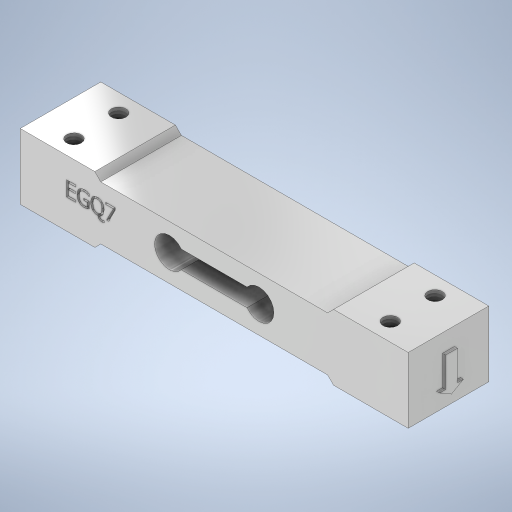
# Autodesk Inventor part: HCMUTE-CDT23-LOADCELL
Saved by Autodesk Inventor 2023 (Build 270158000, 158)
## iProperties
Created: 2023-10-10
Part Number: HCMUTE-CDT23-LOADCELL
Material: Aluminum 6061
Document SubType Name: Modeling
Designer: havie
Density: 2.7 g/cm^3
Appearance: Aluminum - Polished
Author: havie
Autodesk Inventor part; units mm, degrees
note: some values were not read from the file. Chosen so that the rebuilt part matches the saved one: direction of "Emboss1".
ref_plane "YZ Plane" through (0, 0, 0) normal (1, 0, 0) x (0, 1, 0)
ref_plane "XZ Plane" through (0, 0, 0) normal (0, 1, 0) x (-1, 0, 0)
ref_plane "XY Plane" through (0, 0, 0) normal (0, 0, 1) x (1, 0, 0)
sketch "Sketch1" plane through (0, 0, 0) normal (0, 0, 1) x (1, 0, 0)
  line L0 (-65, -13.5) -> (65, -13.5)
  line L1 (65, -13.5) -> (65, 13.5)
  line L2 (65, 13.5) -> (-65, 13.5)
  line L3 (-65, 13.5) -> (-65, -13.5)
  line L4 (-65, -13.5) -> (65, 13.5) construction
  line L5 (65, -13.5) -> (-65, 13.5) construction
  point P0 (0, 0)
  dimension "d0" = 27
  dimension "d1" = 130
  constraints: 12 end point, 2 midpoint, 2 parallel, 1 horizontal, 1 perpendicular
  measures "d0" distance between parallel lines of L2 L0
  measures "d1" distance of L1.end L2.end
extrude "Extrusion1" add sketch "Sketch1" along normal mid plane 22
sketch "Sketch2" plane through (0, 0, 11) normal (0, 0, 1) x (1, 0, 0)
  line L0 (-65, -13.5) -> (65, -13.5) projected
  line L1 (65, -13.5) -> (65, 13.5) projected
  line L2 (-65, 13.5) -> (-65, -13.5) projected
  point P0 (0, 0)
  point P1 (-53, -7.5)
  point P2 (-53, 7.5)
  point P3 (53, 7.5)
  point P4 (53, -7.5)
  dimension "d4" = 6
  dimension "d5" = 15
  dimension "d6" = 12
  dimension "d7" = 12
  constraints: 2 horizontal alignment, 2 vertical alignment
  measures "d4" distance from line of point (53, -7.5) L0
  measures "d5" distance of point (53, 7.5) point (53, -7.5)
  measures "d6" distance from line of L1 point (53, -7.5)
  measures "d7" distance from line of point (-53, -7.5) L2
hole "Hole1" at (-53, -7.5, 11) at (-53, 7.5, 11) at (53, 7.5, 11) at (53, -7.5, 11) direction (0, 0, -1) diameter 4.917 end through all thread size "M6x1" class "6H" standard "ISO Metric profile"
sketch "Sketch3" plane through (-65, -13.5, 11) normal (0, -1, 0) x (1, 0, 0)
  line L0 (0, 0) -> (130, 0) projected
  line L1 (25, 0) -> (27, -2)
  line L2 (27, -2) -> (103, -2)
  line L3 (103, -2) -> (105, 0)
  point P0 (65, -11)
  dimension "d15" = 25
  dimension "d16" = 25
  dimension "d17" = 2
  dimension "d18" = 135
  constraints: 6 end point, 2 point on line, 1 parallel, 1 perpendicular
  measures "d15" distance of L0.start L1.start
  measures "d16" distance of L3.end L0.end
  measures "d17" distance between parallel lines of L0 L2
  measures "d18" angle of L2 L1
extrude "Extrusion2" cut sketch "Sketch3" against normal through all
mirror "Mirror1" about plane through (0, 0, 0) normal (0, 0, 1) of "Extrusion2"
sketch "Sketch4" plane through (65, -13.5, -11) normal (0, -1, 0) x (1, 0, 0)
  circle A0 centre (-80, 11) radius 5
  circle A1 centre (-50, 11) radius 5
  line L0 (-25, 22) -> (0, 22) projected
  line L1 (-76, 14) -> (-54, 14)
  line L2 (-76, 8) -> (-54, 8)
  point P0 (-65, 11)
  dimension "d21" = 10
  dimension "d22" = 10
  dimension "d23" = 30
  dimension "d24" = 15
  dimension "d25" = 11
  dimension "d26" = 6
  dimension "d27" = 3
  constraints: 4 end point, 4 point on circle, 2 centre point, 2 horizontal, 1 horizontal alignment
  measures "d21" diameter of A0
  measures "d22" diameter of A1
  measures "d23" distance of A1.centre A0.centre
  measures "d24" distance of point (-65, 11) A0.centre
  measures "d25" distance from line of L0 A1.centre
  measures "d26" distance between parallel lines of L2 L1
  measures "d27" distance from line of L1 point (-65, 11)
extrude "Extrusion3" cut sketch "Sketch4" against normal through all
sketch "Sketch5" plane through (65, -13.5, 11) normal (1, 0, 0) x (0, 0, -1)
  line L0 (6, 11.5) -> (16, 11.5)
  line L1 (16, 11.5) -> (16, 15.5)
  line L2 (16, 15.5) -> (6, 15.5)
  line L3 (6, 15.5) -> (6, 11.5)
  line L4 (16, 0) -> (16, 27) projected
  line L5 (16, 9.5) -> (18.3094, 13.5)
  line L6 (18.3094, 13.5) -> (16, 17.5)
  line L7 (16, 9.5) -> (16, 17.5)
  point P0 (11, 13.5)
  point P1 (11, 15.5)
  point P2 (16, 11.5)
  dimension "d30" = 4
  dimension "d31" = 2
  dimension "d32" = 10
  dimension "d33" = 5
  dimension "d34" = 8
  dimension "d35" = 2
  dimension "d36" = 30
  constraints: 14 end point, 2 parallel, 2 point on line, 1 collinear, 1 horizontal, 1 horizontal alignment, 1 midpoint, 1 perpendicular
  measures "d30" distance from line of point (11, 15.5) L0
  measures "d31" distance from line of L0 point (11, 13.5)
  measures "d32" distance of L1.end L2.end
  measures "d33" distance from line of point (11, 13.5) L3
  measures "d34" distance of L5.start L6.end
  measures "d35" distance from line of L6.end L2
  measures "d36" angle of L1 L5
extrude "Extrusion4" add sketch "Sketch5" along normal blind 1
sketch "Sketch6" plane through (65, -13.5, -11) normal (0, -1, 0) x (1, 0, 0)
  line L0 (-115, 15) -> (-100, 15) construction
  line L1 (-100, 15) -> (-100, 5) construction
  line L2 (-100, 5) -> (-115, 5) construction
  line L3 (-115, 5) -> (-115, 15) construction
  line L4 (-130, 0) -> (-130, 22) projected
  line L5 (-105, 0) -> (-130, 0) projected
  line L6 (-114.4935, 9.8947) -> (-114.4935, 14.8947)
  line L7 (-114.4935, 14.8947) -> (-111.3655, 14.8947)
  line L8 (-111.3655, 14.8947) -> (-111.3655, 14.3031)
  line L9 (-111.3655, 14.3031) -> (-113.829, 14.3031)
  line L10 (-113.829, 14.3031) -> (-113.829, 12.9335)
  line L11 (-113.829, 12.9335) -> (-111.5316, 12.9335)
  line L12 (-111.5316, 12.9335) -> (-111.5316, 12.342)
  line L13 (-111.5316, 12.342) -> (-113.829, 12.342)
  line L14 (-113.829, 12.342) -> (-113.829, 10.4862)
  line L15 (-113.829, 10.4862) -> (-111.3655, 10.4862)
  line L16 (-111.3655, 10.4862) -> (-111.3655, 9.8947)
  line L17 (-111.3655, 9.8947) -> (-114.4935, 9.8947)
  spline S0 degree 2 poles (-108.5413, 9.7974) (-109.0721, 9.7974) (-109.9514, 10.1216) (-110.2674, 10.4498) knots 0 0 0 1 2 2 2
  spline S1 degree 2 poles (-110.2674, 10.4498) (-110.5835, 10.782) (-110.9198, 11.7626) (-110.9198, 12.3987) knots 0 0 0 1 2 2 2
  spline S2 degree 2 poles (-110.9198, 12.3987) (-110.9198, 13.0024) (-110.5794, 13.9587) (-110.2634, 14.299) knots 0 0 0 1 2 2 2
  spline S3 degree 2 poles (-110.2634, 14.299) (-109.9595, 14.6272) (-109.0681, 14.9838) (-108.5373, 14.9838) knots 0 0 0 1 2 2 2
  spline S4 degree 2 poles (-108.5373, 14.9838) (-108.282, 14.9838) (-107.8201, 14.9109) (-107.6094, 14.846) knots 0 0 0 1 2 2 2
  spline S5 degree 2 poles (-107.6094, 14.846) (-107.4392, 14.7974) (-107.0259, 14.6191) (-106.9003, 14.5543) knots 0 0 0 1 2 2 2
  line L18 (-106.9003, 14.5543) -> (-106.9003, 13.752)
  line L19 (-106.9003, 13.752) -> (-106.9571, 13.752)
  spline S6 degree 2 poles (-106.9571, 13.752) (-107.0827, 13.8614) (-107.346, 14.06) (-107.5891, 14.1734) knots 0 0 0 1 2 2 2
  spline S7 degree 2 poles (-107.5891, 14.1734) (-107.7917, 14.2747) (-108.3144, 14.4084) (-108.6143, 14.4084) knots 0 0 0 1 2 2 2
  spline S8 degree 2 poles (-108.6143, 14.4084) (-109.3355, 14.4084) (-110.2269, 13.3225) (-110.2269, 12.419) knots 0 0 0 1 2 2 2
  spline S9 degree 2 poles (-110.2269, 12.419) (-110.2269, 11.9165) (-109.9919, 11.1629) (-109.769, 10.9036) knots 0 0 0 1 2 2 2
  spline S10 degree 2 poles (-109.769, 10.9036) (-109.5543, 10.6442) (-108.9465, 10.3728) (-108.5656, 10.3728) knots 0 0 0 1 2 2 2
  spline S11 degree 2 poles (-108.5656, 10.3728) (-108.2861, 10.3728) (-107.7269, 10.4538) (-107.5365, 10.5348) knots 0 0 0 1 2 2 2
  line L20 (-107.5365, 10.5348) -> (-107.5365, 11.8274)
  line L21 (-107.5365, 11.8274) -> (-108.6953, 11.8274)
  line L22 (-108.6953, 11.8274) -> (-108.6953, 12.4109)
  line L23 (-108.6953, 12.4109) -> (-106.8801, 12.4109)
  line L24 (-106.8801, 12.4109) -> (-106.8801, 10.2269)
  spline S12 degree 2 poles (-106.8801, 10.2269) (-107.0057, 10.1702) (-107.4352, 9.9959) (-107.6175, 9.9433) knots 0 0 0 1 2 2 2
  spline S13 degree 2 poles (-107.6175, 9.9433) (-107.8647, 9.8703) (-108.2618, 9.7974) (-108.5413, 9.7974) knots 0 0 0 1 2 2 2
  spline S14 degree 2 poles (-101.8922, 8.671) (-102.0746, 8.6264) (-102.4716, 8.5778) (-102.6702, 8.5778) knots 0 0 0 1 2 2 2
  spline S15 degree 2 poles (-102.6702, 8.5778) (-103.2334, 8.5778) (-103.9344, 9.2058) (-103.9668, 9.7893) knots 0 0 0 1 2 2 2
  spline S16 degree 2 poles (-103.9668, 9.7893) (-104.0113, 9.7893) (-104.0883, 9.7893) (-104.1207, 9.7893) knots 0 0 0 1 2 2 2
  spline S17 degree 2 poles (-104.1207, 9.7893) (-104.6272, 9.7893) (-105.4417, 10.1337) (-105.7334, 10.47) knots 0 0 0 1 2 2 2
  spline S18 degree 2 poles (-105.7334, 10.47) (-106.0211, 10.8023) (-106.329, 11.7747) (-106.329, 12.3906) knots 0 0 0 1 2 2 2
  spline S19 degree 2 poles (-106.329, 12.3906) (-106.329, 13.0227) (-106.017, 13.9789) (-105.7293, 14.3193) knots 0 0 0 1 2 2 2
  spline S20 degree 2 poles (-105.7293, 14.3193) (-105.4376, 14.6556) (-104.6232, 15) (-104.1207, 15) knots 0 0 0 1 2 2 2
  spline S21 degree 2 poles (-104.1207, 15) (-103.6102, 15) (-102.7917, 14.6434) (-102.5081, 14.3193) knots 0 0 0 1 2 2 2
  spline S22 degree 2 poles (-102.5081, 14.3193) (-102.2245, 13.9911) (-101.9084, 13.0146) (-101.9084, 12.3906) knots 0 0 0 1 2 2 2
  spline S23 degree 2 poles (-101.9084, 12.3906) (-101.9084, 11.4182) (-102.6661, 10.154) (-103.3266, 9.9311) knots 0 0 0 1 2 2 2
  spline S24 degree 2 poles (-103.3266, 9.9311) (-103.3104, 9.7447) (-103.2131, 9.4449) (-103.1361, 9.3598) knots 0 0 0 1 2 2 2
  spline S25 degree 2 poles (-103.1361, 9.3598) (-103.0429, 9.2545) (-102.7877, 9.1572) (-102.5608, 9.1572) knots 0 0 0 1 2 2 2
  spline S26 degree 2 poles (-102.5608, 9.1572) (-102.4271, 9.1572) (-102.0624, 9.2423) (-101.9814, 9.2747) knots 0 0 0 1 2 2 2
  line L25 (-101.9814, 9.2747) -> (-101.8922, 9.2747)
  line L26 (-101.8922, 9.2747) -> (-101.8922, 8.671)
  spline S27 degree 2 poles (-102.6013, 12.3906) (-102.6013, 12.889) (-102.816, 13.6548) (-103.0105, 13.906) knots 0 0 0 1 2 2 2
  spline S28 degree 2 poles (-103.0105, 13.906) (-103.2091, 14.1653) (-103.7682, 14.4246) (-104.1167, 14.4246) knots 0 0 0 1 2 2 2
  spline S29 degree 2 poles (-104.1167, 14.4246) (-104.4773, 14.4246) (-105.0203, 14.1734) (-105.2269, 13.906) knots 0 0 0 1 2 2 2
  spline S30 degree 2 poles (-105.2269, 13.906) (-105.4254, 13.6507) (-105.6361, 12.8768) (-105.6361, 12.3906) knots 0 0 0 1 2 2 2
  spline S31 degree 2 poles (-105.6361, 12.3906) (-105.6361, 11.406) (-104.8096, 10.3566) (-104.1167, 10.3566) knots 0 0 0 1 2 2 2
  spline S32 degree 2 poles (-104.1167, 10.3566) (-103.4238, 10.3566) (-102.6013, 11.406) (-102.6013, 12.3906) knots 0 0 0 1 2 2 2
  line L27 (-98.1807, 14.1451) -> (-100.3444, 9.8947)
  line L28 (-100.3444, 9.8947) -> (-101.0575, 9.8947)
  line L29 (-101.0575, 9.8947) -> (-98.7723, 14.3071)
  line L30 (-98.7723, 14.3071) -> (-101.3533, 14.3071)
  line L31 (-101.3533, 14.3071) -> (-101.3533, 14.8947)
  line L32 (-101.3533, 14.8947) -> (-98.1807, 14.8947)
  line L33 (-98.1807, 14.8947) -> (-98.1807, 14.1451)
  point P0 (-65, 11)
  dimension "d39" = 15
  dimension "d40" = 5
  dimension "d41" = 15
  dimension "d42" = 10
  constraints: 2 other
  measures "d39" distance between parallel lines of L4 L3
  measures "d40" distance between parallel lines of L5 L2
  measures "d41" distance of L1.end L2.end
  measures "d42" distance of L0.end L1.end
emboss "Emboss1" sketch "Sketch6" operation cut depth 1 direction (0, 1, 0)
body "Solid1"
